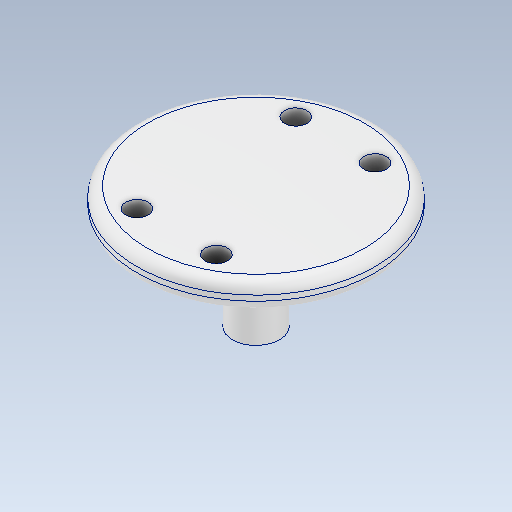
# Autodesk Inventor part: mountingnema
Saved by Autodesk Inventor 2025.1 (Build 291241000, 241)
## iProperties
Created: 2024-11-07
Part Number: mountingnema
Material: Aluminum 6061
Document SubType Name: Modeling
Designer: ramad
Density: 2.7 g/cm^3
Appearance: Aluminum - Flat
Author: ramad
Autodesk Inventor part; units mm, degrees
ref_plane "YZ Plane" through (0, 0, 0) normal (1, 0, 0) x (0, 1, 0)
ref_plane "XZ Plane" through (0, 0, 0) normal (0, 1, 0) x (-1, 0, 0)
ref_plane "XY Plane" through (0, 0, 0) normal (0, 0, 1) x (1, 0, 0)
sketch "Sketch1" plane through (0, 0, 0) normal (0, 1, 0) x (-1, 0, 0)
  circle A0 centre (0, 0) radius 4.45
  circle A1 centre (0, 0) radius 2.55
  dimension "d0" = 8.9
  dimension "d1" = 5.1
  constraints: 2 centre point, 2 coincident
  measures "d0" diameter of A0
  measures "d1" diameter of A1
extrude "Extrusion1" add sketch "Sketch1" along normal blind 18
sketch "Sketch2" plane through (0, 18, 0) normal (0, 1, 0) x (1, 0, 0)
  line L0 (25, -25) -> (-25, -25)
  line L1 (-25, -25) -> (-25, 25)
  line L2 (-25, 25) -> (25, 25)
  line L3 (25, 25) -> (25, -25)
  line L4 (25, -25) -> (-25, 25) construction
  line L5 (-25, -25) -> (25, 25) construction
  line L6 (7.5, -12.875) -> (-7.5, -12.875)
  line L7 (-7.5, -12.875) -> (-7.5, 12.875)
  line L8 (-7.5, 12.875) -> (7.5, 12.875)
  line L9 (7.5, 12.875) -> (7.5, -12.875)
  line L10 (7.5, -12.875) -> (-7.5, 12.875) construction
  line L11 (-7.5, -12.875) -> (7.5, 12.875) construction
  line L12 (-7.5, 12.875) -> (-7.5, 17.125)
  circle A0 centre (-7.5, 15) radius 2.125
  circle A1 centre (7.5, 15) radius 2.125
  line L13 (-7.5, -12.875) -> (-7.5, -17.125)
  circle A2 centre (-7.5, -15) radius 2.125
  circle A3 centre (7.5, -15) radius 2.125
  circle A4 centre (0, 0) radius 4.45 projected
  circle A5 centre (0, 0) radius 22.5
  dimension "d7" = 50
  dimension "d8" = 50
  dimension "d9" = 15
  dimension "d10" = 25.75
  dimension "d11" = 4.25
  dimension "d12" = 4.25
  dimension "d13" = 45
  constraints: 28 end point, 4 midpoint, 4 parallel, 4 vertical alignment, 2 centre point, 2 horizontal, 2 perpendicular, 2 vertical, 1 coincident, 6 other
  measures "d7" distance of L1.end L2.end
  measures "d8" distance of L0.end L1.end
  measures "d9" distance of L7.end L8.end
  measures "d10" distance of L6.end L7.end
  measures "d11" distance of L7.end L12.end
  measures "d12" distance of L6.end L13.end
  measures "d13" diameter of A5
extrude "Extrusion2" add sketch "Sketch2" along normal blind 5 contours L6 L7 L8 L9 | A4 | A5
fillet "Fillet1" radius 2 2 edges at (-22.5, 18, 0) (-22.5, 23, 0)
body "Solid1"
